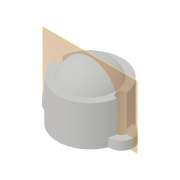
# Autodesk Inventor part: CasterBallTemp
Saved by Autodesk Inventor 2018 (Build 220112000, 112)
## iProperties
Created: 2019-02-16
Part Number: CasterBallTemp
Material: Generic
Document SubType Name: Modeling
Designer: ball
Density: 1 g/cm^3
Appearance: Default
Author: ball
Autodesk Inventor part; units mm, degrees
ref_plane "YZ Plane" through (0, 0, 0) normal (1, 0, 0) x (0, 1, 0)
ref_plane "XZ Plane" through (0, 0, 0) normal (0, 1, 0) x (-1, 0, 0)
sketch "Sketch1" plane through (0, 0, 0) normal (0, 0, 1) x (1, 0, 0)
  arc A0 (6.35, 7.112) -> (-6.35, 7.112) centre (0, 7.112) ccw
  line L0 (-6.35, 7.112) -> (6.35, 7.112)
  point P0 (0, 0)
  dimension "d0" = 12.7
  constraints: 2 end point, 2 point on circle, 1 centre point, 1 horizontal
  measures "d0" diameter of A0
revolve "Revolution1" add sketch "Sketch1" angle 360 about axis through (-6.35, 7.112, 0) along (1, 0, 0)
sketch "Sketch2" plane through (0, 0, 0) normal (0, 1, 0) x (-1, 0, 0)
  circle A0 centre (0, 0) radius 7.62
  dimension "d2" = 15.24
  constraints: 1 centre point, 1 coincident
  measures "d2" diameter of A0
extrude "Extrusion1" add sketch "Sketch2" along normal blind 9.398
sketch "Sketch4" plane through (0, 0, 0) normal (0, -1, 0) x (1, 0, 0)
  arc A0 (-7.62, 0) -> (-7.62, 0) centre (7.366, 0) ccw projected
  circle A1 centre (7.366, 0) radius 2.794
  arc A2 (-7.62, 0) -> (-7.62, 0) centre (-7.366, 0) ccw projected
  circle A3 centre (-7.366, 0) radius 2.794
  point P0 (0, 0)
  dimension "d9" = 5.588
  dimension "d10" = 5.588
  constraints: 2 centre point, 2 coincident, 2 other
  measures "d9" diameter of A1
  measures "d10" diameter of A3
extrude "Extrusion3" add sketch "Sketch4" against normal blind 2.032 contours A2 | A3 A0 | A0 A3 | A1 picked at (-6.7956, 1.0953) picked at (-8.3961, -0.643)
sketch "Sketch5" plane through (0, 0, 0) normal (0, -1, 0) x (1, 0, 0)
  circle A0 centre (-7.366, 0) radius 1.143
  circle A1 centre (7.366, 0) radius 1.143
  point P0 (0, 0)
  dimension "d13" = 2.286
  dimension "d14" = 2.286
  constraints: 2 centre point, 2 coincident
  measures "d13" diameter of A0
  measures "d14" diameter of A1
extrude "Extrusion4" cut sketch "Sketch5" against normal through all
body "Solid1"
